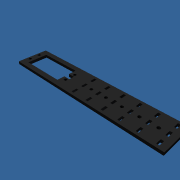
# Autodesk Inventor part: Acrylic_UpperArm
Saved by Autodesk Inventor 2012 (Build 160160000, 160)
## iProperties
Created: 2014-03-29
Part Number: Acrylic_UpperArm
Material: Default
Document SubType Name: Modeling
Designer: Admin
Density: 1 g/cm^3
Author: Admin
Autodesk Inventor part; units mm, degrees
ref_plane "YZ Plane" through (0, 0, 0) normal (1, 0, 0) x (0, 1, 0)
ref_plane "XZ Plane" through (0, 0, 0) normal (0, 1, 0) x (-1, 0, 0)
ref_plane "XY Plane" through (0, 0, 0) normal (0, 0, 1) x (1, 0, 0)
sketch "Sketch1" plane through (0, 0, 0) normal (0, 0, 1) x (1, 0, 0)
  line L0 (-30, -18) -> (-30, 12)
  line L1 (-30, 12) -> (120, 12)
  line L2 (120, 12) -> (120, -18)
  line L3 (120, -18) -> (-30, -18)
  point P0 (-30, -3)
  dimension "d13" = 30
  dimension "d55" = 150
  constraints: 8 end point, 1 horizontal, 1 midpoint, 1 parallel, 1 perpendicular, 1 other
  measures "d13" distance of L1.end L2.end
  measures "d55" distance of L2.end L0.start
extrude "Extrusion1" add sketch "Sketch1" along normal blind 2.8
sketch "Sketch4" plane through (0, 0, 2.8) normal (0, 0, 1) x (1, 0, 0)
  line L0 (-22.4, 6.9) -> (17.9, 6.9)
  line L1 (17.9, -0.5) -> (23.9, -0.5)
  line L2 (17.9, -12.9) -> (-22.4, -12.9)
  line L3 (17.9, -5.5) -> (17.9, -12.9)
  line L4 (17.9, -5.5) -> (17.9, -12.9)
  line L5 (23.9, -5.5) -> (17.9, -5.5)
  line L6 (-22.4, -12.9) -> (-22.4, 6.9)
  line L7 (23.9, -0.5) -> (23.9, -5.5)
  line L8 (17.9, 6.9) -> (17.9, -0.5)
  circle A0 centre (-26.75, -8) radius 2.5
  circle A1 centre (-26.75, 2) radius 2.5
  circle A2 centre (22.25, -8) radius 2.5
  circle A3 centre (22.25, 2) radius 2.5
  circle A4 centre (22.25, -8) radius 1.5
  circle A5 centre (22.25, 2) radius 1.5
  circle A6 centre (-26.75, -8) radius 1.5
  circle A7 centre (-26.75, 2) radius 1.5
  line L9 (120, 12) -> (120, -18) projected
  line L10 (-30, -18) -> (-30, 12) projected
  line L11 (120, -18) -> (-30, -18) projected
  line L12 (120, -3) -> (-30, -3)
  line L13 (112.8, -0.5) -> (115, -0.5)
  line L14 (115, -0.5) -> (115, -5.5)
  line L15 (115, -5.5) -> (112.8, -5.5)
  line L16 (112.8, -5.5) -> (112.8, -0.5)
  line L17 (97.8, -0.5) -> (100, -0.5)
  line L18 (100, -0.5) -> (100, -5.5)
  line L19 (100, -5.5) -> (97.8, -5.5)
  line L20 (97.8, -5.5) -> (97.8, -0.5)
  line L21 (82.8, -0.5) -> (85, -0.5)
  line L22 (85, -0.5) -> (85, -5.5)
  line L23 (85, -5.5) -> (82.8, -5.5)
  line L24 (82.8, -5.5) -> (82.8, -0.5)
  line L25 (67.8, -0.5) -> (70, -0.5)
  line L26 (70, -0.5) -> (70, -5.5)
  line L27 (70, -5.5) -> (67.8, -5.5)
  line L28 (67.8, -5.5) -> (67.8, -0.5)
  line L29 (52.8, -0.5) -> (55, -0.5)
  line L30 (55, -0.5) -> (55, -5.5)
  line L31 (55, -5.5) -> (52.8, -5.5)
  line L32 (52.8, -5.5) -> (52.8, -0.5)
  line L33 (37.8, -0.5) -> (40, -0.5)
  line L34 (40, -0.5) -> (40, -5.5)
  line L35 (40, -5.5) -> (37.8, -5.5)
  line L36 (37.8, -5.5) -> (37.8, -0.5)
  line L37 (112.8, -10.5) -> (115, -10.5)
  line L38 (115, -10.5) -> (115, -15.5)
  line L39 (115, -15.5) -> (112.8, -15.5)
  line L40 (112.8, -15.5) -> (112.8, -10.5)
  line L41 (97.8, -10.5) -> (100, -10.5)
  line L42 (100, -10.5) -> (100, -15.5)
  line L43 (100, -15.5) -> (97.8, -15.5)
  line L44 (97.8, -15.5) -> (97.8, -10.5)
  line L45 (82.8, -10.5) -> (85, -10.5)
  line L46 (85, -10.5) -> (85, -15.5)
  line L47 (85, -15.5) -> (82.8, -15.5)
  line L48 (82.8, -15.5) -> (82.8, -10.5)
  line L49 (67.8, -10.5) -> (70, -10.5)
  line L50 (70, -10.5) -> (70, -15.5)
  line L51 (70, -15.5) -> (67.8, -15.5)
  line L52 (67.8, -15.5) -> (67.8, -10.5)
  line L53 (52.8, -10.5) -> (55, -10.5)
  line L54 (55, -10.5) -> (55, -15.5)
  line L55 (55, -15.5) -> (52.8, -15.5)
  line L56 (52.8, -15.5) -> (52.8, -10.5)
  line L57 (37.8, -10.5) -> (40, -10.5)
  line L58 (40, -10.5) -> (40, -15.5)
  line L59 (40, -15.5) -> (37.8, -15.5)
  line L60 (37.8, -15.5) -> (37.8, -10.5)
  line L61 (112.8, 9.5) -> (112.8, 4.5)
  line L62 (115, 4.5) -> (115, 9.5)
  line L63 (115, 9.5) -> (112.8, 9.5)
  line L64 (112.8, 4.5) -> (115, 4.5)
  line L65 (97.8, 9.5) -> (97.8, 4.5)
  line L66 (100, 4.5) -> (100, 9.5)
  line L67 (100, 9.5) -> (97.8, 9.5)
  line L68 (97.8, 4.5) -> (100, 4.5)
  line L69 (82.8, 9.5) -> (82.8, 4.5)
  line L70 (85, 4.5) -> (85, 9.5)
  line L71 (85, 9.5) -> (82.8, 9.5)
  line L72 (82.8, 4.5) -> (85, 4.5)
  line L73 (67.8, 9.5) -> (67.8, 4.5)
  line L74 (70, 4.5) -> (70, 9.5)
  line L75 (70, 9.5) -> (67.8, 9.5)
  line L76 (67.8, 4.5) -> (70, 4.5)
  line L77 (52.8, 9.5) -> (52.8, 4.5)
  line L78 (55, 4.5) -> (55, 9.5)
  line L79 (55, 9.5) -> (52.8, 9.5)
  line L80 (52.8, 4.5) -> (55, 4.5)
  line L81 (37.8, 9.5) -> (37.8, 4.5)
  line L82 (40, 4.5) -> (40, 9.5)
  line L83 (40, 9.5) -> (37.8, 9.5)
  line L84 (37.8, 4.5) -> (40, 4.5)
  circle A8 centre (106.4, -3) radius 1.5
  circle A9 centre (91.4, -3) radius 1.5
  circle A10 centre (76.4, -3) radius 1.5
  circle A11 centre (61.4, -3) radius 1.5
  circle A12 centre (46.4, -3) radius 1.5
  dimension "d51" = 3
  dimension "d52" = 3
  dimension "d53" = 3
  dimension "d54" = 3
  dimension "d56" = 2.2
  dimension "d57" = 5
  dimension "d58" = 2.5
  dimension "d59" = 5
  dimension "d62" = 15
  dimension "d65" = 10
  dimension "d68" = 3
  dimension "d69" = 6.4
  dimension "d72" = 15
  constraints: 164 end point, 24 symmetric about line, 13 centre point, 7 horizontal, 6 vertical, 4 coincident, 2 midpoint, 2 parallel, 1 perpendicular, 1 point on line, 112 other
  measures "d51" diameter of A4
  measures "d52" diameter of A5
  measures "d53" diameter of A6
  measures "d54" diameter of A7
  measures "d56" distance of L14.end L15.end
  measures "d57" distance of L13.end L14.end
  measures "d58" distance between parallel lines of L12 L13
  measures "d59" distance between parallel lines of L9 L14
  measures "d62" distance of L13.start L20.end
  measures "d65" distance of L13.start L40.end
  measures "d68" diameter of A8
  measures "d69" distance from line of L16 A8.centre
  measures "d72" distance of A8.centre A9.centre
extrude "Extrusion3" cut sketch "Sketch4" against normal blind 10 contours L0 L8 L1 L7 L12 L6 | L12 L7 L5 L3 L2 L6 | L36 L33 L34 L12 | L12 L34 L35 L36 | A12 L12 | L12 A12 | L14 L15 L16 L12 | L12 L16 L13 L14 | L32 L29 L30 L12 | L12 L30 L31 L32 | A8 L12 | L12 A8 | A11 L12 | L12 A11 | L18 L19 L20 L12 | L12 L20 L17 L18 | L28 L25 L26 L12 | L12 L26 L27 L28 | A9 L12 | L12 A9 | A10 L12 | L12 A10 | L22 L23 L24 L12 | L12 L24 L21 L22 | A4 | A5 | A6 | A7 | L37 L38 L39 L40 | L41 L42 L43 L44 | L45 L46 L47 L48 | L49 L50 L51 L52 | L53 L54 L55 L56 | L57 L58 L59 L60 | L63 L62 L64 L61 | L67 L66 L68 L65 | L71 L70 L72 L69 | L75 L74 L76 L73 | L79 L78 L80 L77 | L83 L82 L84 L81
body "Solid1"
